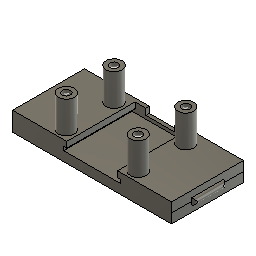
Login_base v6 (Autodesk Fusion 360 design; units mm, degrees)
Autodesk Fusion 360 part; units mm, degrees
sketch "Sketch6" plane through (0, -2.041031, 0) normal (0, -1, 0) x (1, 0, 0)
  arc A0 (-8.867818, -6.766526) -> (-6.867818, -8.766526) centre (-6.867818, -6.766526) ccw
  line L0 (-6.867818, -8.766526) -> (6.932182, -8.766526)
  arc A1 (6.932182, -8.766526) -> (8.932182, -6.766526) centre (6.932182, -6.766526) ccw
  line L1 (8.932182, -6.766526) -> (8.932182, -6.686526)
  line L2 (8.932182, -6.686526) -> (7.652182, -6.686526)
  arc A2 (7.652182, -4.886526) -> (7.652182, -6.686526) centre (7.652182, -5.786526) ccw
  line L3 (7.652182, -4.886526) -> (8.932182, -4.886526)
  line L4 (8.932182, -4.886526) -> (8.932182, -4.146526)
  line L5 (8.932182, -4.146526) -> (7.652182, -4.146526)
  arc A3 (7.652182, -2.346526) -> (7.652182, -4.146526) centre (7.652182, -3.246526) ccw
  line L6 (7.652182, -2.346526) -> (8.932182, -2.346526)
  line L7 (8.932182, -2.346526) -> (8.932182, -1.606526)
  line L8 (8.932182, -1.606526) -> (7.652182, -1.606526)
  arc A4 (7.652182, 0.193474) -> (7.652182, -1.606526) centre (7.652182, -0.706526) ccw
  line L9 (7.652182, 0.193474) -> (8.932182, 0.193474)
  line L10 (8.932182, 0.193474) -> (8.932182, 0.933474)
  line L11 (8.932182, 0.933474) -> (7.652182, 0.933474)
  arc A5 (7.652182, 2.733474) -> (7.652182, 0.933474) centre (7.652182, 1.833474) ccw
  line L12 (7.652182, 2.733474) -> (8.932182, 2.733474)
  line L13 (8.932182, 2.733474) -> (8.932182, 3.473474)
  line L14 (8.932182, 3.473474) -> (7.652182, 3.473474)
  arc A6 (7.652182, 5.273474) -> (7.652182, 3.473474) centre (7.652182, 4.373474) ccw
  line L15 (7.652182, 5.273474) -> (8.932182, 5.273474)
  line L16 (8.932182, 5.273474) -> (8.932182, 6.013474)
  line L17 (8.932182, 6.013474) -> (7.652182, 6.013474)
  arc A7 (7.652182, 7.813474) -> (7.652182, 6.013474) centre (7.652182, 6.913474) ccw
  line L18 (7.652182, 7.813474) -> (8.932182, 7.813474)
  line L19 (8.932182, 7.813474) -> (8.932182, 8.553474)
  line L20 (8.932182, 8.553474) -> (7.652182, 8.553474)
  arc A8 (7.652182, 10.353474) -> (7.652182, 8.553474) centre (7.652182, 9.453474) ccw
  line L21 (7.652182, 10.353474) -> (8.932182, 10.353474)
  line L22 (8.932182, 10.353474) -> (8.932182, 10.433474)
  arc A9 (8.932182, 10.433474) -> (6.932182, 12.433474) centre (6.932182, 10.433474) ccw
  line L23 (6.932182, 12.433474) -> (-6.867818, 12.433474)
  arc A10 (-6.867818, 12.433474) -> (-8.867818, 10.433474) centre (-6.867818, 10.433474) ccw
  line L24 (-8.867818, 10.433474) -> (-8.867818, 10.353474)
  line L25 (-8.867818, 10.353474) -> (-7.587818, 10.353474)
  arc A11 (-7.587818, 8.553474) -> (-7.587818, 10.353474) centre (-7.587818, 9.453474) ccw
  line L26 (-7.587818, 8.553474) -> (-8.867818, 8.553474)
  line L27 (-8.867818, 8.553474) -> (-8.867818, 7.813474)
  line L28 (-8.867818, 7.813474) -> (-7.587818, 7.813474)
  arc A12 (-7.587818, 6.013474) -> (-7.587818, 7.813474) centre (-7.587818, 6.913474) ccw
  line L29 (-7.587818, 6.013474) -> (-8.867818, 6.013474)
  line L30 (-8.867818, 6.013474) -> (-8.867818, 5.273474)
  line L31 (-8.867818, 5.273474) -> (-7.587818, 5.273474)
  arc A13 (-7.587818, 3.473474) -> (-7.587818, 5.273474) centre (-7.587818, 4.373474) ccw
  line L32 (-7.587818, 3.473474) -> (-8.867818, 3.473474)
  line L33 (-8.867818, 3.473474) -> (-8.867818, 2.733474)
  line L34 (-8.867818, 2.733474) -> (-7.587818, 2.733474)
  arc A14 (-7.587818, 0.933474) -> (-7.587818, 2.733474) centre (-7.587818, 1.833474) ccw
  line L35 (-7.587818, 0.933474) -> (-8.867818, 0.933474)
  line L36 (-8.867818, 0.933474) -> (-8.867818, 0.193474)
  line L37 (-8.867818, 0.193474) -> (-7.587818, 0.193474)
  arc A15 (-7.587818, -1.606526) -> (-7.587818, 0.193474) centre (-7.587818, -0.706526) ccw
  line L38 (-7.587818, -1.606526) -> (-8.867818, -1.606526)
  line L39 (-8.867818, -1.606526) -> (-8.867818, -2.346526)
  line L40 (-8.867818, -2.346526) -> (-7.587818, -2.346526)
  arc A16 (-7.587818, -4.146526) -> (-7.587818, -2.346526) centre (-7.587818, -3.246526) ccw
  line L41 (-7.587818, -4.146526) -> (-8.867818, -4.146526)
  line L42 (-8.867818, -4.146526) -> (-8.867818, -4.886526)
  line L43 (-8.867818, -4.886526) -> (-7.587818, -4.886526)
  arc A17 (-7.587818, -6.686526) -> (-7.587818, -4.886526) centre (-7.587818, -5.786526) ccw
  line L44 (-7.587818, -6.686526) -> (-8.867818, -6.686526)
  line L45 (-8.867818, -6.686526) -> (-8.867818, -6.766526)
  line L46 (0.032182, -8.766526) -> (0.032182, 12.433474)
  line L47 (25.032182, 12.533474) -> (-24.967818, 12.533474)
  line L48 (-24.967818, 12.533474) -> (-24.967818, -8.866526)
  line L49 (-24.967818, -8.866526) -> (25.032182, -8.866526)
  line L50 (25.032182, -8.866526) -> (25.032182, 12.533474)
  line L51 (25.032182, 12.533474) -> (-24.967818, -8.866526) construction
  line L52 (-24.967818, 12.533474) -> (25.032182, -8.866526) construction
  point P0 (0.032182, 1.833474)
  point P1 (0.032182, 1.833474)
  dimension "d1" = 50
  dimension "d2" = 21.4
  constraint horizontal L47
  constraint perpendicular L47 L48
  constraint parallel L47 L49
  constraint parallel L48 L50
extrude "Extrude1" add sketch "Sketch6" along normal blind 3 contours A0 L0 L23 A10 L24 L25 A11 L26 L27 L28 A12 L29 L30 L31 A13 L32 L33 L34 A14 L35 L36 L37 A15 L38 L39 L40 A16 L41 L42 L43 A17 L44 L45 L46 | L0 A1 L1 L2 A2 L3 L4 L5 A3 L6 L7 L8 A4 L9 L10 L11 A5 L12 L13 L14 A6 L15 L16 L17 A7 L18 L19 L20 A8 L21 L22 A9 L23 L46 | L47 L48 L49 L50 picked at (-2.208657, 1.811055) picked at (2.273021, 1.855893) picked at (-19.601151, 2.133474) makes body 1
sketch "Sketch7" plane through (0, 0, 12.533474) normal (0, 0, 1) x (1, 0, 0)
  line L0 (25.032182, -2.041031) -> (-24.967818, -2.041031)
  line L1 (-24.967818, -2.041031) -> (-24.967818, -5.041031)
  line L2 (-24.967818, -5.041031) -> (25.032182, -5.041031)
  line L3 (25.032182, -5.041031) -> (25.032182, -2.041031)
  line L4 (-8.867843, -2.041031) -> (8.932257, -2.041031)
  line L5 (15.032207, -2.041031) -> (15.032207, 0.958969)
  line L6 (-14.967793, 0.958969) -> (-14.967793, -2.041031)
  line L7 (8.982207, -0.891031) -> (8.982207, -2.041031)
  line L8 (-8.917793, -2.041031) -> (-8.917793, -0.891031)
  line L9 (15.032207, 0.958969) -> (8.032207, 0.958969)
  line L10 (-7.967793, 0.958969) -> (-14.967793, 0.958969)
  line L11 (-8.917793, -0.891031) -> (-7.967793, -0.891031)
  line L12 (8.032207, -0.891031) -> (8.982207, -0.891031)
  line L13 (-7.967793, -1.013098) -> (-7.967793, 0.958969)
  line L14 (8.032207, 0.958969) -> (8.032207, -0.891031)
  line L15 (-14.967793, -2.041031) -> (15.032207, -2.041031)
  point P0 (0.032207, -2.041031)
  point P1 (0.032207, -2.041031)
  point P2 (0.032207, -2.041031)
  dimension "d5" = 17.8001
  dimension "d6" = 30
  constraint parallel L0 L4
  constraint parallel L5 L6
  constraint horizontal L11
  constraint perpendicular L7 L11
  constraint parallel L7 L8
  constraint collinear L9 L10
  constraint collinear L11 L12
  constraint perpendicular L5 L15
extrude "Extrude2" add sketch "Sketch7" against normal blind 21.4 contours L0 L5 L7 L9 L12 L14 L15 | L0 L6 L8 L10 L11 L13 L15 picked at (13.015541, -0.657698) picked at (-12.951126, -0.657698) bodies 1
extrude "Extrude3" add 1 faces at (15.032207, -1.041031, 5.40014) along direction (1, 0, 0) blind 10 on bodies 1 bodies 1
extrude "Extrude4" add 1 faces at (-14.967793, -0.041031, 5.40014) along direction (-1, 0, 0) blind 10 on bodies 1 bodies 1
sketch "Sketch8" plane through (0, 0.958969, 0) normal (0, 1, 0) x (-1, 0, 0)
  line L0 (-8.032207, 12.533474) -> (-25.032207, 12.533474)
  line L1 (-25.032207, 12.533474) -> (-25.032207, -8.866526)
  line L2 (-25.032207, -8.866526) -> (-8.032207, -8.866526)
  line L3 (-8.032207, -8.866526) -> (-8.032207, 12.533474)
  line L4 (24.967793, 12.533474) -> (24.967793, -8.866526)
  line L5 (-25.032207, 1.833474) -> (24.967793, 1.833474)
  line L6 (-11.332207, 9.333474) -> (11.267793, -5.666526) construction
  line L7 (11.267793, 9.333474) -> (-11.332207, -5.666526) construction
  circle A0 centre (11.267793, -5.666526) radius 2.5
  circle A1 centre (-11.332207, -5.666526) radius 2.5
  circle A2 centre (11.267793, 9.333474) radius 2.5
  circle A3 centre (-11.332207, 9.333474) radius 2.5
  point P0 (30, -14)
  point P1 (24.967793, 1.833474)
  point P2 (-25.032207, 1.833474)
  point P3 (-0.032207, 1.833474)
  point P4 (-0.032207, 1.833474)
  dimension "d17" = 22.6
  dimension "d18" = 15
  dimension "d19" = 5
  dimension "d22" = -22.6
  dimension "d23" = 15
  measures "d19" diameter of A0
extrude "Extrude5" add sketch "Sketch8" along normal blind 10 contours A0 | A1 | A2 | A3 picked at (11.082359, -4.92751) picked at (-11.517641, -4.92751) picked at (9.869381, 9.178596) picked at (-12.730619, 9.178596) bodies 1
sketch "Sketch9" plane through (0, 10.958969, 0) normal (0, 1, 0) x (-1, 0, 0)
  circle A0 centre (11.267793, -5.666526) radius 2.5
  circle A1 centre (11.267793, -5.666526) radius 2.5
  point P0 (-11.332207, -5.666526)
  point P1 (11.267793, 9.333474)
  point P2 (-11.332207, 9.333474)
  dimension "d28" = -22.6
  dimension "d29" = 15
  constraint concentric A0 A1
hole "Hole1" at (-11.267793, 10.958969, -5.666526) at (-11.267793, 10.958969, 9.333474) at (11.332207, 10.958969, 9.333474) at (11.332207, 10.958969, -5.666526) direction (0, -1, 0) diameter 2.529 depth 8 tip angle 180 bodies 1
thread "Thread1" "ISO Metric profile 3.0 M3x0.5 6H" thread offset 1 thread depth 7
extrude "Extrude6" add 1 faces at (3.015524, -4.041031, -8.866526) along direction (0, 0, -1) blind 1.2 on bodies 1 bodies 1
sketch "Sketch10" plane through (0, 0, -10.066526) normal (0, 0, -1) x (-1, 0, 0)
  line L0 (24.967818, -2.041031) -> (24.967793, -2.041031)
  line L1 (24.967793, -2.041031) -> (24.967793, 0.958969)
  line L2 (24.967793, 0.958969) -> (7.967793, 0.958969)
  line L3 (7.967793, 0.958969) -> (7.967793, -0.891031)
  line L4 (7.967793, -0.891031) -> (8.917793, -0.891031)
  line L5 (8.917793, -0.891031) -> (8.917793, -2.041031)
  line L6 (8.917793, -2.041031) -> (-8.982207, -2.041031)
  line L7 (-8.982207, -2.041031) -> (-8.982207, -0.891031)
  line L8 (-8.982207, -0.891031) -> (-8.032207, -0.891031)
  line L9 (-8.032207, -0.891031) -> (-8.032207, 0.958969)
  line L10 (-8.032207, 0.958969) -> (-25.032207, 0.958969)
  line L11 (-25.032207, 0.958969) -> (-25.032207, -2.041031)
  line L12 (-25.032207, -2.041031) -> (-25.032182, -2.041031)
  line L13 (-25.032182, -2.041031) -> (-25.032182, -5.041031)
  line L14 (-25.032182, -5.041031) -> (24.967818, -5.041031)
  line L15 (24.967818, -5.041031) -> (24.967818, -2.041031)
  line L16 (7.967793, -0.891031) -> (8.917793, -0.891031)
  line L17 (8.917793, -2.041031) -> (-8.982207, -2.041031)
  line L18 (-8.982207, -0.891031) -> (-8.032207, -0.891031)
  line L19 (-4.6, -1) -> (4.535585, -1)
  line L20 (4.535585, -1) -> (4.535585, 0.958969)
  line L21 (-4.6, 0.958969) -> (-4.6, -1)
  line L22 (-8.032207, 0.958969) -> (-4.6, 0.958969)
  line L23 (4.535585, 0.958969) -> (7.967793, 0.958969)
  constraint horizontal L19
  constraint perpendicular L19 L20
  constraint parallel L20 L21
  constraint collinear L22 L23
extrude "Extrude7" add sketch "Sketch10" against normal blind 1.1 contours L3 L4 L5 L6 L7 L8 L9 L16 L17 L18 L19 L20 L21 L22 L23 picked at (-5.744069, -0.310687) bodies 1
sketch "Sketch11" plane through (25.032207, 0, 0) normal (1, 0, 0) x (0, 0, -1)
  line L0 (-12.533474, 0.958969) -> (-12.533474, -2.041031)
  line L1 (-12.533474, -2.041031) -> (10.066526, -2.041031)
  line L2 (10.066526, -2.041031) -> (10.066526, 0.958969)
  line L3 (10.066526, 0.958969) -> (-12.533474, 0.958969)
  line L4 (-12.533474, -2.041031) -> (10.066526, -2.041031)
  line L5 (3.766526, -1.041031) -> (-6.233474, -1.041031)
  line L6 (-6.233474, -1.041031) -> (-6.233474, -3.041031)
  line L7 (-6.233474, -3.041031) -> (3.766526, -3.041031)
  line L8 (3.766526, -3.041031) -> (3.766526, -1.041031)
  line L9 (3.766526, -1.041031) -> (-6.233474, -3.041031) construction
  line L10 (-6.233474, -1.041031) -> (3.766526, -3.041031) construction
  point P0 (-1.233474, -2.041031)
  point P1 (-1.233474, -2.041031)
  dimension "d43" = 10
  dimension "d44" = 2
  constraint horizontal L5
  constraint perpendicular L5 L6
  constraint parallel L5 L7
  constraint parallel L6 L8
extrude "Extrude8" add sketch "Sketch11" along normal blind 1 contours L1 L4 L5 L6 L8 | L1 L4 L6 L7 L8 picked at (0.433193, -1.707698) picked at (-2.90014, -2.374364) bodies 1
fillet "Fillet1" radius 1 4 edges at (26.032207, -1.041031, 1.233474) (26.032207, -3.041031, 1.233474) (26.032207, -2.041031, 6.233474) (26.032207, -2.041031, -3.766526) on bodies 1
sketch "Sketch12" plane through (-24.967793, 0, 0) normal (-1, 0, 0) x (0, 0, 1)
  line L0 (12.533474, -2.041031) -> (12.533474, 0.958969)
  line L1 (12.533474, 0.958969) -> (-10.066526, 0.958969)
  line L2 (-10.066526, 0.958969) -> (-10.066526, -2.041031)
  line L3 (-10.066526, -2.041031) -> (12.533474, -2.041031)
  line L4 (-10.066526, -2.041031) -> (12.533474, -2.041031)
  line L5 (-3.766526, -3.041031) -> (6.233474, -3.041031)
  line L6 (6.233474, -3.041031) -> (6.233474, -1.041031)
  line L7 (6.233474, -1.041031) -> (-3.766526, -1.041031)
  line L8 (-3.766526, -1.041031) -> (-3.766526, -3.041031)
  line L9 (-3.766526, -3.041031) -> (6.233474, -1.041031) construction
  line L10 (6.233474, -3.041031) -> (-3.766526, -1.041031) construction
  point P0 (1.233474, -2.041031)
  point P1 (1.233474, -2.041031)
  dimension "d49" = 10
  dimension "d50" = 2
  constraint horizontal L5
  constraint perpendicular L5 L6
  constraint parallel L5 L7
  constraint parallel L6 L8
extrude "Extrude9" add sketch "Sketch12" along normal blind 1 separate body contours L3 L4 L5 L6 L8 | L3 L4 L6 L7 L8 picked at (2.90014, -2.374364) picked at (-0.433193, -1.374364) makes body 2
fillet "Fillet2" radius 1 4 edges at (-25.967793, -2.041031, -3.766526) (-25.967793, -1.041031, 1.233474) (-25.967793, -3.041031, 1.233474) (-25.967793, -2.041031, 6.233474) on bodies 2
